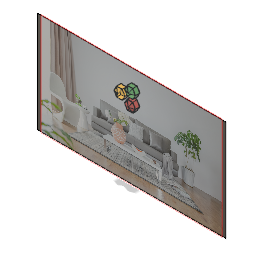
22-Day 16 - Hexagonal Wall Mounted Rack v1 (Autodesk Fusion 360 design; units mm, degrees)
Autodesk Fusion 360 part; units mm, degrees
note: some values were not read from the file. Set by a fixed rule: which sketch regions a step uses.
sketch "Sketch1" plane through (0, 0, 0) normal (0, 0, 1) x (1, 0, 0)
  line L0 (0, 50) -> (-43.3013, 25)
  line L1 (-43.3013, 25) -> (-43.3013, -25)
  line L2 (-43.3013, -25) -> (0, -50)
  line L3 (0, -50) -> (43.3013, -25)
  line L4 (43.3013, -25) -> (43.3013, 25)
  line L5 (43.3013, 25) -> (0, 50)
  line L6 (-45.3013, -26.1547) -> (0, -52.3094)
  line L7 (0, -52.3094) -> (45.3013, -26.1547)
  line L8 (45.3013, -26.1547) -> (45.3013, 26.1547)
  line L9 (45.3013, 26.1547) -> (0, 52.3094)
  line L10 (0, 52.3094) -> (-45.3013, 26.1547)
  line L11 (-45.3013, 26.1547) -> (-45.3013, -26.1547)
  dimension "d1" = 2
extrude "Extrude1" add sketch "Sketch1" along normal blind 2 contours L0 L1 L2 L3 L4 L5 | L6 L7 L8 L9 L10 L11 makes body 1
extrude "Extrude2" add sketch "Sketch1" along normal blind 40 bodies 1
move_body "Move1" bodies 1 to x (0, 1, 0) y (-1, 0, 0) z (0, 0, 1) at (0, 0, 0)
ref_plane "WorkPlane2" through (0, 45.3013, 20) normal (0, 1, 0) x (-1, 0, 0)
ref_plane "WorkPlane3" through (39.2321, 22.6506, 20) normal (0.866025, 0.5, 0) x (-0.5, 0.866025, 0)
mirror "Mirror1" about plane through (39.2321, 22.6506, 20) normal (0.866025, 0.5, 0) of bodies 1 makes body 2
mirror "Mirror2" about plane through (0, 45.3013, 20) normal (0, 1, 0) of bodies 1 makes body 3
ref_plane "WorkPlane4" through (0, 90.6025, 40) normal (0, 0, 1) x (0, -1, 0)
sketch "Sketch3" plane through (0, 90.6025, 40) normal (0, 0, 1) x (1, 0, 0)
  line L0 (-25, -43.3013) -> (-50, 0)
  line L1 (-50, 0) -> (-25, 43.3013)
  line L2 (-25, 43.3013) -> (25, 43.3013)
  line L3 (25, 43.3013) -> (50, 0)
  line L4 (50, 0) -> (25, -43.3013)
  line L5 (25, -43.3013) -> (-25, -43.3013)
  line L6 (26.1547, 45.3013) -> (-26.1547, 45.3013)
  line L7 (-26.1547, 45.3013) -> (-52.3094, 0)
  line L8 (-52.3094, 0) -> (-26.1547, -45.3013)
  line L9 (-26.1547, -45.3013) -> (26.1547, -45.3013)
  line L10 (26.1547, -45.3013) -> (52.3094, 0)
  line L11 (52.3094, 0) -> (26.1547, 45.3013)
  line L12 (-26.1547, 45.3013) -> (-25, 43.3013)
  line L13 (25, -43.3013) -> (26.1547, -45.3013)
  constraint coincident L6.end L7.start
  constraint coincident L9.end L10.start
  constraint collinear L12 L13
extrude "Extrude3" add sketch "Sketch3" along normal blind 20 separate body makes body 4
chamfer "Chamfer1" distance 45 distance2 20 6 edges at (-39.2321, 113.2532, 60) (0, 135.9038, 60) (39.2321, 113.2532, 60) (39.2321, 67.9519, 60) (0, 45.3013, 60) (-39.2321, 67.9519, 60) measured on face at (0, 90.6025, 60) measured on face at (0, 90.6025, 60) measured on face at (0, 90.6025, 60) measured on face at (0, 90.6025, 60) measured on face at (0, 90.6025, 60) measured on face at (0, 90.6025, 60) on bodies 4
shell "Shell1" thickness 2 removed faces 1 at (0, 90.6025, 40) on bodies 4
mirror "Mirror3" about plane through (0, 45.3013, 20) normal (0, 1, 0) of bodies 4 makes body 5
mirror "Mirror4" about plane through (39.2321, 22.6506, 20) normal (0.866025, 0.5, 0) of bodies 5 makes body 6
sketch "Sketch4" plane through (0, 90.6025, 40) normal (0, 0, 1) x (1, 0, 0)
  line L0 (0.1739, -0.3013) -> (-0.1739, -0.3013)
  line L1 (-0.1739, -0.3013) -> (-26.1547, -45.3013)
  line L2 (-26.1547, -45.3013) -> (26.1547, -45.3013)
  line L3 (26.1547, -45.3013) -> (0.1739, -0.3013)
  line L4 (78.2902, -45.6025) -> (78.1162, -45.3013)
  line L5 (78.1162, -45.3013) -> (26.1547, -45.3013)
  line L6 (26.1547, -45.3013) -> (52.3094, -90.6025)
  line L7 (52.3094, -90.6025) -> (78.2902, -45.6025)
  line L8 (-26.1547, -135.9038) -> (26.1547, -135.9038)
  line L9 (26.1547, -135.9038) -> (0.1739, -90.9038)
  line L10 (0.1739, -90.9038) -> (-0.1739, -90.9038)
  line L11 (-0.1739, -90.9038) -> (-26.1547, -135.9038)
  line L12 (-26.1547, 45.3013) -> (52.3094, -90.6025)
  line L13 (26.1547, -45.3013) -> (-26.1547, -135.9038)
  line L14 (78.1162, -45.3013) -> (78.2902, -45)
  line L15 (78.2902, -45) -> (52.3094, 0)
  line L16 (52.3094, 0) -> (26.1547, -45.3013)
  line L17 (26.1547, -45.3013) -> (78.1162, -45.3013)
  line L18 (26.1547, -45.3013) -> (52.3094, 0)
  line L19 (-26.1547, -135.9038) -> (-100, -135.9038)
  line L20 (-26.1547, 45.3013) -> (-100, 45.3013)
  line L21 (-100, 45.3013) -> (-100, -135.9038)
  line L22 (-26.1547, 45.3013) -> (26.1547, -45.3013)
  line L23 (52.3094, 0) -> (154.8835, 0)
  line L24 (52.3094, -90.6025) -> (154.8835, -90.6025)
  line L25 (154.8835, -90.6025) -> (154.8835, 0)
  line L26 (52.3094, 0) -> (78.2902, -45.6025)
  line L27 (52.3094, -90.6025) -> (104.6188, -90.6025)
  line L28 (104.6188, -90.6025) -> (78.638, -45.6025)
  line L29 (78.638, -45.6025) -> (78.2902, -45.6025)
  line L30 (78.2902, -45.6025) -> (52.3094, -90.6025)
  line L31 (52.3094, 0) -> (104.6188, -90.6025)
  line L32 (-26.1547, 45.3013) -> (50, 45.3013)
  line L33 (50, 45.3013) -> (52.3094, 0)
  line L34 (104.6188, -90.6025) -> (52.3094, -90.6025)
  line L35 (78.638, -45) -> (104.6188, 0)
  line L36 (78.4641, -45.3013) -> (104.6188, 0)
  line L37 (0.1739, 0.3013) -> (26.1547, 45.3013)
  line L38 (-0.1739, -0.3013) -> (26.1547, 45.3013)
  point P0 (-26.1547, 45.3013)
  constraint coincident P0 L12.start
  constraint coincident L6.end L7.start
  constraint coincident L2.end L3.start
  constraint coincident L8.start L11.end
  constraint coincident L15.end L16.start
  constraint parallel L8 L19
  constraint parallel L19 L20
  constraint perpendicular L19 L21
  constraint parallel L5 L23
  constraint parallel L23 L24
  constraint perpendicular L23 L25
  constraint coincident L4.start L7.end
  constraint coincident L27.end L28.start
  constraint parallel L20 L32
  constraint midpoint L31 L36.start
  constraint coincident L35.end L36.end
  constraint coincident L0.end L1.start
  constraint coincident L37.end L38.end
extrude "Extrude5" cut sketch "Sketch4" along normal blind 50 contours L0 L1 L2 L3 L12 L22 | L3 L12 L16 L18 L22 L32 L33 L37 L38 | L5 L16 L17 L18 L26 | L4 L5 L6 L7 L12 L17 L26 L30 | L7 L24 L27 L28 L29 L30 L31 L34 bodies 4 6
sketch "Sketch5" plane through (0, 90.6025, 40) normal (0, 0, 1) x (1, 0, 0)
  line L0 (100, -90) -> (-100, -90)
  line L1 (-0.1739, -90.3013) -> (0.1739, -90.3013)
  line L2 (0.1739, -90.3013) -> (26.1547, -45.3013)
  line L3 (26.1547, -45.3013) -> (-26.1547, -45.3013)
  line L4 (-26.1547, -45.3013) -> (-0.1739, -90.3013)
  line L5 (-26.1547, -45.3013) -> (-100, -45.3013)
  line L6 (-100, -45.3013) -> (-26.1547, -45.3013)
  line L7 (69.2533, -45.3013) -> (-26.1547, -45.3013)
  line L8 (69.2533, -45.3013) -> (69.2533, -90)
  line L9 (-100, -45.3013) -> (-100, -90)
  constraint horizontal L0
  constraint coincident L3.end L4.start
  constraint parallel L3 L5
  constraint parallel L3 L7
  constraint coincident L0 L8.end
  constraint perpendicular L0 L8
  constraint perpendicular L0 L9
extrude "Extrude6" cut sketch "Sketch5" along normal blind 60 contours L0 L2 L7 L8 | L0 L2 L3 L4 L7 | L0 L4 L5 L6 L9 keep common part bodies 5
combine "Combine1" operation add target body 4 tool bodies 3
combine "Combine2" operation add target body 2 tool bodies 6
combine "Combine3" operation add target body 1 tool bodies 5
move_body "Align1" bodies 1 to x (1, 0, 0) y (0, 1, 0) z (0, 0, 1) at (78.4641, 135.9038, 0)
move_body "Move5" bodies 2 to x (1, 0, 0) y (0, 1, 0) z (0, 0, 1) at (0, -60, 0)
move_body "Align2" bodies 2 to x (1, 0, 0) y (0, 1, 0) z (0, 0, 1) at (-78.4641, 14.6987, 0)
move_body "Align3" bodies 2 to x (1, 0, 0) y (0, 1, 0) z (0, 0, 1) at (-78.4641, 135.9038, 0)
move_body "Align4" bodies 2 to x (1, 0, 0) y (0, 1, 0) z (0, 0, 1) at (156.9282, -90.6025, 0)
move_body "Move6" bodies 4 to x (1, 0, 0) y (0, 1, 0) z (0, 0, 1) at (-10, 0, 0)
move_body "Move7" bodies 1 to x (1, 0, 0) y (0, 1, 0) z (0, 0, 1) at (0, 5, 0)
move_body "Move8" bodies 2 to x (1, 0, 0) y (0, 1, 0) z (0, 0, 1) at (0, -5, 0)
move_body "Move9" bodies 4 to x (1, 0, 0) y (0, 1, 0) z (0, 0, 1) at (-10, 0, 0)
move_body "Move10" bodies 1 to x (1, 0, 0) y (0, 1, 0) z (0, 0, 1) at (0, 5, 0)
move_body "Move11" bodies 2 to x (1, 0, 0) y (0, 1, 0) z (0, 0, 1) at (0, -5, 0)
sketch "Sketch6" plane through (0, 0, 0) normal (0, 0, 1) x (1, 0, 0)
  line L0 (-700, 400) -> (700, 400)
  line L1 (700, 400) -> (700, -350)
  line L2 (700, -350) -> (-700, -350)
  line L3 (-700, -350) -> (-700, 400)
  constraint horizontal L0
  constraint vertical L1
  constraint horizontal L2
  constraint vertical L3
extrude "Extrude7" add sketch "Sketch6" against normal blind 2 separate body makes body 7
move_body "Move12" bodies 4 1 2 to x (1, 0, 0) y (0, 1, 0) z (0, 0, 1) at (0, 110, 0)
move_body "Move13" bodies 1 4 2 to x (1, 0, 0) y (0, 1, 0) z (0, 0, 1) at (-20, 30, 0)
scale "Scale1" factor 0.8 about (-92.3094, 230.6025, 40) bodies 4 1 2
